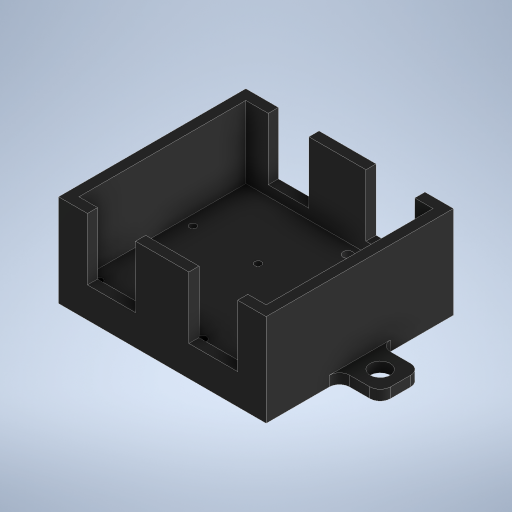
# Autodesk Inventor part: pololuAndRelayCaseBottom
Saved by Autodesk Inventor 2024 (Build 280153000, 153)
## iProperties
Created: 2023-08-11
Part Number: pololuAndRelayCaseBottom
Material: Rubber, Silicone
Document SubType Name: Modeling
Designer: 18179
Density: 1.25 g/cm^3
Appearance: Rubber - Black
Autodesk Inventor part; units mm, degrees
ref_plane "YZ Plane" through (0, 0, 0) normal (1, 0, 0) x (0, 1, 0)
ref_plane "XZ Plane" through (0, 0, 0) normal (0, 1, 0) x (-1, 0, 0)
ref_plane "XY Plane" through (0, 0, 0) normal (0, 0, 1) x (1, 0, 0)
sketch "0" plane through (0, 0, 0) normal (0, 0, 1) x (1, 0, 0)
  line L0 (-1.8843, 38.1841) -> (-1.8843, 30.5641)
  line L1 (-1.8843, 30.5641) -> (-4.4243, 30.5641)
  line L2 (-4.4243, 30.5641) -> (-4.4243, 38.1841)
  line L3 (-4.4243, 38.1841) -> (-1.8843, 38.1841)
  line L4 (0, 50.8) -> (-25.4, 50.8)
  line L5 (-25.4, 50.8) -> (-25.4, 0)
  line L6 (-25.4, 0) -> (0, 0)
  line L7 (0, 0) -> (0, 50.8)
  line L8 (-20.2946, 10.414) -> (-20.2946, 28.194)
  line L9 (-20.2946, 28.194) -> (-5.1054, 28.194)
  line L10 (-5.1054, 28.194) -> (-5.1054, 10.414)
  line L11 (-5.1054, 10.414) -> (-5.08, 10.414)
  line L12 (-5.08, 10.414) -> (-5.08, 2.667)
  line L13 (-5.08, 2.667) -> (-20.32, 2.667)
  line L14 (-20.32, 2.667) -> (-20.32, 10.414)
  line L15 (-20.32, 10.414) -> (-20.2946, 10.414)
  line L16 (-20.32, 41.275) -> (-20.32, 49.022)
  line L17 (-20.32, 49.022) -> (-5.08, 49.022)
  line L18 (-5.08, 49.022) -> (-5.08, 41.275)
  line L19 (-5.08, 41.275) -> (-20.32, 41.275)
  circle A0 centre (-22.733, 2.5852) radius 1.524
  circle A1 centre (-2.667, 2.5852) radius 1.524
  circle A2 centre (-22.733, 48.2148) radius 1.524
  circle A3 centre (-2.667, 48.2148) radius 1.524
  line L20 (-51.95, 5.718) -> (-51.95, 1.218)
  line L21 (-36.95, 1.218) -> (-51.95, 1.218)
  line L22 (-36.95, 5.718) -> (-36.95, 1.218)
  line L23 (-36.95, 5.718) -> (-51.95, 5.718)
  circle A4 centre (-39.45, 3.468) radius 1.775
  circle A5 centre (-44.45, 3.468) radius 1.775
  circle A6 centre (-49.45, 3.468) radius 1.775
  line L24 (-36.95, 7.268) -> (-51.95, 7.268)
  circle A7 centre (-34.29, 2.54) radius 1.0922
  circle A8 centre (-54.61, 2.54) radius 1.0922
  circle A9 centre (-54.61, 31.75) radius 1.0922
  circle A10 centre (-34.29, 31.75) radius 1.0922
  line L25 (-48.655, 31.516) -> (-48.28, 32.141)
  line L26 (-48.28, 32.141) -> (-48.24, 32.141)
  line L27 (-48.24, 32.141) -> (-47.865, 31.516)
  line L28 (-47.865, 31.516) -> (-46.115, 31.516)
  line L29 (-46.115, 31.516) -> (-45.74, 32.141)
  line L30 (-45.74, 32.141) -> (-45.7, 32.141)
  line L31 (-45.7, 32.141) -> (-45.325, 31.516)
  line L32 (-45.325, 31.516) -> (-43.575, 31.516)
  line L33 (-43.575, 31.516) -> (-43.2, 32.141)
  line L34 (-43.2, 32.141) -> (-43.16, 32.141)
  line L35 (-43.16, 32.141) -> (-42.785, 31.516)
  line L36 (-42.785, 31.516) -> (-41.035, 31.516)
  line L37 (-41.035, 31.516) -> (-40.66, 32.141)
  line L38 (-40.66, 32.141) -> (-40.62, 32.141)
  line L39 (-40.62, 32.141) -> (-40.245, 31.516)
  line L40 (-40.245, 31.516) -> (-38.495, 31.516)
  line L41 (-38.495, 31.516) -> (-38.12, 32.141)
  line L42 (-38.12, 32.141) -> (-38.1, 32.141)
  line L43 (-38.1, 32.141) -> (-38.1, 33.391)
  line L44 (-38.1, 33.391) -> (-38.12, 33.391)
  line L45 (-38.12, 33.391) -> (-38.495, 34.016)
  line L46 (-38.495, 34.016) -> (-40.245, 34.016)
  line L47 (-40.245, 34.016) -> (-40.62, 33.391)
  line L48 (-40.62, 33.391) -> (-40.66, 33.391)
  line L49 (-40.66, 33.391) -> (-41.035, 34.016)
  line L50 (-41.035, 34.016) -> (-42.785, 34.016)
  line L51 (-42.785, 34.016) -> (-43.16, 33.391)
  line L52 (-43.16, 33.391) -> (-43.2, 33.391)
  line L53 (-43.2, 33.391) -> (-43.575, 34.016)
  line L54 (-43.575, 34.016) -> (-45.325, 34.016)
  line L55 (-45.325, 34.016) -> (-45.7, 33.391)
  line L56 (-45.7, 33.391) -> (-45.74, 33.391)
  line L57 (-45.74, 33.391) -> (-46.115, 34.016)
  line L58 (-46.115, 34.016) -> (-47.865, 34.016)
  line L59 (-47.865, 34.016) -> (-48.24, 33.391)
  line L60 (-48.24, 33.391) -> (-48.28, 33.391)
  line L61 (-48.28, 33.391) -> (-48.655, 34.016)
  line L62 (-48.655, 34.016) -> (-50.405, 34.016)
  line L63 (-50.405, 34.016) -> (-50.78, 33.391)
  line L64 (-50.78, 33.391) -> (-50.8, 33.391)
  line L65 (-50.8, 33.391) -> (-50.8, 32.141)
  line L66 (-50.8, 32.141) -> (-50.78, 32.141)
  line L67 (-50.78, 32.141) -> (-50.405, 31.516)
  line L68 (-50.405, 31.516) -> (-48.655, 31.516)
  line L69 (-49.205, 32.441) -> (-49.205, 33.091)
  line L70 (-49.205, 32.441) -> (-49.855, 32.441)
  line L71 (-49.855, 32.441) -> (-49.855, 33.091)
  line L72 (-49.205, 33.091) -> (-49.855, 33.091)
  line L73 (-44.125, 32.441) -> (-44.125, 33.091)
  line L74 (-44.125, 32.441) -> (-44.775, 32.441)
  line L75 (-44.775, 32.441) -> (-44.775, 33.091)
  line L76 (-44.125, 33.091) -> (-44.775, 33.091)
  line L77 (-39.045, 32.441) -> (-39.045, 33.091)
  line L78 (-39.045, 32.441) -> (-39.695, 32.441)
  line L79 (-39.695, 32.441) -> (-39.695, 33.091)
  line L80 (-39.045, 33.091) -> (-39.695, 33.091)
  line L81 (-41.585, 32.441) -> (-41.585, 33.091)
  line L82 (-41.585, 32.441) -> (-42.235, 32.441)
  line L83 (-42.235, 32.441) -> (-42.235, 33.091)
  line L84 (-41.585, 33.091) -> (-42.235, 33.091)
  line L85 (-46.665, 32.441) -> (-46.665, 33.091)
  line L86 (-46.665, 32.441) -> (-47.315, 32.441)
  line L87 (-47.315, 32.441) -> (-47.315, 33.091)
  line L88 (-46.665, 33.091) -> (-47.315, 33.091)
  line L89 (-31.75, 34.29) -> (-57.15, 34.29)
  line L90 (-57.15, 34.29) -> (-57.15, 0)
  line L91 (-57.15, 0) -> (-31.75, 0)
  line L92 (-31.75, 0) -> (-31.75, 34.29)
  line L93 (-43.3742, 24.6136) -> (-43.3742, 24.6236)
  line L94 (-43.3742, 24.6236) -> (-42.8742, 24.6236)
  line L95 (-42.8742, 24.6236) -> (-42.8742, 24.6136)
  line L96 (-43.3742, 24.6136) -> (-42.8742, 24.6136)
  line L97 (-42.4242, 24.6136) -> (-42.4242, 24.6236)
  line L98 (-42.4242, 24.6236) -> (-41.9242, 24.6236)
  line L99 (-41.9242, 24.6236) -> (-41.9242, 24.6136)
  line L100 (-42.4242, 24.6136) -> (-41.9242, 24.6136)
  line L101 (-41.4742, 24.6136) -> (-41.4742, 24.6236)
  line L102 (-41.4742, 24.6236) -> (-40.9742, 24.6236)
  line L103 (-40.9742, 24.6236) -> (-40.9742, 24.6136)
  line L104 (-41.4742, 24.6136) -> (-40.9742, 24.6136)
  line L105 (-48.714, 27.3595) -> (-48.714, 27.171)
  line L106 (-48.714, 27.3595) -> (-48.314, 27.3595)
  line L107 (-48.314, 27.3595) -> (-48.314, 27.171)
  line L108 (-48.314, 27.171) -> (-48.714, 27.171)
  line L109 (-48.314, 24.6595) -> (-48.314, 24.848)
  line L110 (-48.714, 24.6595) -> (-48.314, 24.6595)
  line L111 (-48.714, 24.6595) -> (-48.714, 24.848)
  line L112 (-48.714, 24.848) -> (-48.314, 24.848)
  line L113 (-51.0762, 27.3595) -> (-51.0762, 27.171)
  line L114 (-51.0762, 27.3595) -> (-50.6762, 27.3595)
  line L115 (-50.6762, 27.3595) -> (-50.6762, 27.171)
  line L116 (-50.6762, 27.171) -> (-51.0762, 27.171)
  line L117 (-50.6762, 24.6595) -> (-50.6762, 24.848)
  line L118 (-51.0762, 24.6595) -> (-50.6762, 24.6595)
  line L119 (-51.0762, 24.6595) -> (-51.0762, 24.848)
  line L120 (-51.0762, 24.848) -> (-50.6762, 24.848)
  line L121 (-33.109, 6.6231) -> (-33.109, 5.8231)
  line L122 (-33.109, 5.8231) -> (-34.709, 5.8231)
  line L123 (-34.709, 5.8231) -> (-34.709, 6.6231)
  line L124 (-34.709, 6.6231) -> (-33.109, 6.6231)
  line L125 (-47.014, 30.867) -> (-46.714, 30.867)
  line L126 (-46.714, 30.867) -> (-45.614, 30.867)
  line L127 (-45.614, 30.867) -> (-45.314, 30.867)
  line L128 (-45.314, 30.867) -> (-45.314, 29.967)
  line L129 (-45.614, 29.967) -> (-45.314, 29.967)
  line L130 (-45.614, 29.967) -> (-46.714, 29.967)
  line L131 (-47.014, 29.967) -> (-46.714, 29.967)
  line L132 (-47.014, 30.867) -> (-47.014, 29.967)
  line L133 (-47.0018, 29.1022) -> (-46.7018, 29.1022)
  line L134 (-46.7018, 29.1022) -> (-45.6018, 29.1022)
  line L135 (-45.6018, 29.1022) -> (-45.3018, 29.1022)
  line L136 (-45.3018, 29.1022) -> (-45.3018, 28.2022)
  line L137 (-45.6018, 28.2022) -> (-45.3018, 28.2022)
  line L138 (-45.6018, 28.2022) -> (-46.7018, 28.2022)
  line L139 (-47.0018, 28.2022) -> (-46.7018, 28.2022)
  line L140 (-47.0018, 29.1022) -> (-47.0018, 28.2022)
  line L141 (-38.4374, 30.141) -> (-38.4374, 29.041)
  line L142 (-38.4374, 29.041) -> (-38.4374, 28.741)
  line L143 (-38.4374, 28.741) -> (-39.3374, 28.741)
  line L144 (-39.3374, 29.041) -> (-39.3374, 28.741)
  line L145 (-39.3374, 29.041) -> (-39.3374, 30.141)
  line L146 (-39.3374, 30.441) -> (-39.3374, 30.141)
  line L147 (-38.4374, 30.441) -> (-39.3374, 30.441)
  line L148 (-38.4374, 30.441) -> (-38.4374, 30.141)
  line L149 (-34.164, 25.019) -> (-33.654, 25.019)
  line L150 (-34.164, 25.029) -> (-34.164, 25.019)
  line L151 (-34.164, 25.029) -> (-33.654, 25.029)
  line L152 (-33.654, 25.019) -> (-33.654, 25.029)
  line L153 (-34.569, 27.519) -> (-35.079, 27.519)
  line L154 (-34.569, 27.519) -> (-34.569, 27.509)
  line L155 (-34.569, 27.509) -> (-35.079, 27.509)
  line L156 (-35.079, 27.519) -> (-35.079, 27.509)
  line L157 (-32.739, 27.519) -> (-33.249, 27.519)
  line L158 (-32.739, 27.519) -> (-32.739, 27.509)
  line L159 (-32.739, 27.509) -> (-33.249, 27.509)
  line L160 (-33.249, 27.519) -> (-33.249, 27.509)
  line L161 (-48.862, 30.466) -> (-47.912, 30.466)
  line L162 (-47.912, 30.466) -> (-47.912, 28.716)
  line L163 (-47.912, 28.716) -> (-48.862, 28.716)
  line L164 (-48.862, 28.716) -> (-48.862, 30.466)
  line L165 (-40.988, 30.466) -> (-40.038, 30.466)
  line L166 (-40.038, 30.466) -> (-40.038, 28.716)
  line L167 (-40.038, 28.716) -> (-40.988, 28.716)
  line L168 (-40.988, 28.716) -> (-40.988, 30.466)
  line L169 (-42.385, 30.466) -> (-41.435, 30.466)
  line L170 (-41.435, 30.466) -> (-41.435, 28.716)
  line L171 (-41.435, 28.716) -> (-42.385, 28.716)
  line L172 (-42.385, 28.716) -> (-42.385, 30.466)
  line L173 (-37.324, 28.354) -> (-37.324, 29.304)
  line L174 (-37.324, 29.304) -> (-35.574, 29.304)
  line L175 (-35.574, 29.304) -> (-35.574, 28.354)
  line L176 (-35.574, 28.354) -> (-37.324, 28.354)
  line L177 (-50.4114, 30.466) -> (-49.4614, 30.466)
  line L178 (-49.4614, 30.466) -> (-49.4614, 28.716)
  line L179 (-49.4614, 28.716) -> (-50.4114, 28.716)
  line L180 (-50.4114, 28.716) -> (-50.4114, 30.466)
  line L181 (-55.612, 24.671) -> (-55.612, 25.621)
  line L182 (-55.612, 25.621) -> (-53.862, 25.621)
  line L183 (-53.862, 25.621) -> (-53.862, 24.671)
  line L184 (-53.862, 24.671) -> (-55.612, 24.671)
  line L185 (-43.7312, 30.466) -> (-42.7812, 30.466)
  line L186 (-42.7812, 30.466) -> (-42.7812, 28.716)
  line L187 (-42.7812, 28.716) -> (-43.7312, 28.716)
  line L188 (-43.7312, 28.716) -> (-43.7312, 30.466)
  line L189 (-41.4742, 27.558) -> (-40.9742, 27.558)
  line L190 (-40.9742, 27.548) -> (-40.9742, 27.558)
  line L191 (-41.4742, 27.548) -> (-40.9742, 27.548)
  line L192 (-41.4742, 27.558) -> (-41.4742, 27.548)
  line L193 (-42.4242, 27.558) -> (-41.9242, 27.558)
  line L194 (-41.9242, 27.548) -> (-41.9242, 27.558)
  line L195 (-42.4242, 27.548) -> (-41.9242, 27.548)
  line L196 (-42.4242, 27.558) -> (-42.4242, 27.548)
  line L197 (-43.3742, 27.558) -> (-42.8742, 27.558)
  line L198 (-42.8742, 27.548) -> (-42.8742, 27.558)
  line L199 (-43.3742, 27.548) -> (-42.8742, 27.548)
  line L200 (-43.3742, 27.558) -> (-43.3742, 27.548)
  line L201 (-38.9509, 26.6649) -> (-38.9509, 26.1671)
  line L202 (-38.9409, 26.6649) -> (-38.9509, 26.6649)
  line L203 (-38.9409, 26.6649) -> (-38.9409, 26.1671)
  line L204 (-38.9509, 26.1671) -> (-38.9409, 26.1671)
  line L205 (-38.9509, 27.6174) -> (-38.9509, 27.1196)
  line L206 (-38.9409, 27.6174) -> (-38.9509, 27.6174)
  line L207 (-38.9409, 27.6174) -> (-38.9409, 27.1196)
  line L208 (-38.9509, 27.1196) -> (-38.9409, 27.1196)
  line L209 (-38.9509, 25.7124) -> (-38.9509, 25.2146)
  line L210 (-38.9409, 25.7124) -> (-38.9509, 25.7124)
  line L211 (-38.9409, 25.7124) -> (-38.9409, 25.2146)
  line L212 (-38.9509, 25.2146) -> (-38.9409, 25.2146)
  line L213 (-35.9637, 27.6174) -> (-35.9637, 27.1196)
  line L214 (-35.9537, 27.6174) -> (-35.9637, 27.6174)
  line L215 (-35.9537, 27.6174) -> (-35.9537, 27.1196)
  line L216 (-35.9637, 27.1196) -> (-35.9537, 27.1196)
  line L217 (-35.9637, 25.7124) -> (-35.9637, 25.2146)
  line L218 (-35.9537, 25.7124) -> (-35.9637, 25.7124)
  line L219 (-35.9537, 25.7124) -> (-35.9537, 25.2146)
  line L220 (-35.9637, 25.2146) -> (-35.9537, 25.2146)
  line L221 (-45.9984, 27.3304) -> (-46.5084, 27.3304)
  line L222 (-45.9984, 27.3204) -> (-45.9984, 27.3304)
  line L223 (-45.9984, 27.3204) -> (-46.5084, 27.3204)
  line L224 (-46.5084, 27.3304) -> (-46.5084, 27.3204)
  line L225 (-45.5934, 24.8304) -> (-45.0834, 24.8304)
  line L226 (-45.5934, 24.8304) -> (-45.5934, 24.8404)
  line L227 (-45.5934, 24.8404) -> (-45.0834, 24.8404)
  line L228 (-45.0834, 24.8304) -> (-45.0834, 24.8404)
  line L229 (-47.4234, 24.8304) -> (-46.9134, 24.8304)
  line L230 (-47.4234, 24.8304) -> (-47.4234, 24.8404)
  line L231 (-47.4234, 24.8404) -> (-46.9134, 24.8404)
  line L232 (-46.9134, 24.8304) -> (-46.9134, 24.8404)
  circle A11 centre (-53.0606, 27.8892) radius 0.508
  circle A12 centre (-44.45, 3.068) radius 0.889
  circle A13 centre (-39.45, 3.068) radius 0.889
  circle A14 centre (-49.45, 3.068) radius 0.889
  circle A15 centre (-39.37, 32.766) radius 0.508
  circle A16 centre (-55.6006, 27.8892) radius 0.508
  circle A17 centre (-50.324, 21.748) radius 0.762
  circle A18 centre (-38.124, 21.748) radius 0.762
  circle A19 centre (-38.124, 9.748) radius 0.762
  circle A20 centre (-50.324, 9.748) radius 0.762
  circle A21 centre (-52.324, 15.748) radius 0.762
  circle A22 centre (-54.61, 31.75) radius 1.0922
  circle A23 centre (-34.29, 31.75) radius 1.0922
  circle A24 centre (-54.61, 2.54) radius 1.0922
  circle A25 centre (-49.53, 4.826) radius 0.508
  circle A26 centre (-44.45, 4.826) radius 0.508
  circle A27 centre (-41.91, 32.766) radius 0.508
  circle A28 centre (-44.45, 32.766) radius 0.508
  circle A29 centre (-46.99, 32.766) radius 0.508
  circle A30 centre (-49.53, 32.766) radius 0.508
  circle A31 centre (-34.29, 2.54) radius 1.0922
  circle A32 centre (-39.37, 4.826) radius 0.508
  line L233 (-25.4, 0) -> (-31.75, 0)
  line L234 (-31.75, 0) -> (-31.75, 12.7114)
  line L235 (-31.75, 12.7114) -> (-25.4, 12.7114)
  line L236 (-25.4, 12.7114) -> (-25.4, 0)
  point P0 (-57.15, 34.29)
  dimension "d0" = 6.35
  constraints: 474 end point, 33 centre point, 2 parallel, 1 horizontal, 1 perpendicular
  measures "d0" distance of L234.end L235.end
extrude "Extrusion1" add sketch "0" along normal blind 3.175 contours L0 L1 L2 L3 | L7 L6 L5 L4 | L92 L91 L90 L89 | L93 L94 L95 L96 | L97 L98 L99 L100 | L101 L102 L103 L104 | L106 L107 L108 L105 | L110 L111 L112 L109 | L114 L115 L116 L113 | L118 L119 L120 L117 | L121 L122 L123 L124 | L125 L126 L127 L128 L129 L130 L131 L132 | L133 L134 L135 L136 L137 L138 L139 L140 | L141 L142 L143 L144 L145 L146 L147 L148 | L150 L151 L152 L149 | L154 L155 L156 L153 | L161 L162 L163 L164 | L165 L166 L167 L168 | L169 L170 L171 L172 | L173 L174 L175 L176 | L177 L178 L179 L180 | L181 L182 L183 L184 | L185 L186 L187 L188 | L189 L190 L191 L192 | L193 L194 L195 L196 | L197 L198 L199 L200 | L202 L203 L204 L201 | L206 L207 L208 L205 | L210 L211 L212 L209 | L214 L215 L216 L213 | L218 L219 L220 L217 | L222 L223 L224 L221 | L226 L227 L228 L225 | L230 L231 L232 L229 | A11 | A16 | A17 | A18 | A19 | A20 | A21
sketch "Sketch3" plane through (0, 0, 3.175) normal (0, 0, 1) x (1, 0, 0)
  line L0 (-57.15, 34.29) -> (-57.15, 0) projected
  line L1 (0, 0) -> (0, 50.8) projected
  line L2 (-57.15, 0) -> (0, 0)
  line L3 (0, 0) -> (0, 50.8)
  line L4 (0, 50.8) -> (-57.15, 50.8)
  line L5 (-57.15, 50.8) -> (-57.15, 0)
  line L6 (-57.785, 51.435) -> (0.635, 51.435)
  line L7 (0.635, 51.435) -> (0.635, -0.635)
  line L8 (0.635, -0.635) -> (-57.785, -0.635)
  line L9 (-57.785, -0.635) -> (-57.785, 51.435)
  line L10 (3.81, 54.61) -> (-60.96, 54.61)
  line L11 (-60.96, 54.61) -> (-60.96, -3.81)
  line L12 (-60.96, -3.81) -> (3.81, -3.81)
  line L13 (3.81, -3.81) -> (3.81, 54.61)
  dimension "d3" = 0.635
  dimension "d4" = 3.175
  constraints: 24 end point, 6 parallel, 3 perpendicular, 1 horizontal, 6 other
  measures "d3" distance between parallel lines of L4 L6
  measures "d4" distance between parallel lines of L6 L10
extrude "Extrusion2" add sketch "Sketch3" along normal blind 3.175 contours L13 L12 L11 L10
sketch "Sketch4" plane through (0, 0, 6.35) normal (0, 0, 1) x (1, 0, 0)
  line L0 (-31.75, 0) -> (-31.75, 34.29) projected
  line L1 (-31.75, 34.29) -> (-57.15, 34.29) projected
  line L2 (-57.15, 34.29) -> (-57.15, 0) projected
  line L3 (-57.15, 0) -> (-31.75, 0) projected
  line L4 (-36.95, 5.718) -> (-36.95, 1.218) projected
  line L5 (-36.95, 1.218) -> (-51.95, 1.218) projected
  line L6 (-51.95, 1.218) -> (-51.95, 5.718) projected
  line L7 (-51.95, 5.718) -> (-36.95, 5.718) projected
  line L8 (-48.655, 31.516) -> (-50.405, 31.516) projected
  line L9 (-50.405, 31.516) -> (-50.78, 32.141) projected
  line L10 (-50.78, 32.141) -> (-50.8, 32.141) projected
  line L11 (-50.8, 32.141) -> (-50.8, 33.391) projected
  line L12 (-50.8, 33.391) -> (-50.78, 33.391) projected
  line L13 (-50.78, 33.391) -> (-50.405, 34.016) projected
  line L14 (-50.405, 34.016) -> (-48.655, 34.016) projected
  line L15 (-48.655, 34.016) -> (-48.28, 33.391) projected
  line L16 (-48.28, 33.391) -> (-48.24, 33.391) projected
  line L17 (-48.24, 33.391) -> (-47.865, 34.016) projected
  line L18 (-47.865, 34.016) -> (-46.115, 34.016) projected
  line L19 (-46.115, 34.016) -> (-45.74, 33.391) projected
  line L20 (-45.74, 33.391) -> (-45.7, 33.391) projected
  line L21 (-45.7, 33.391) -> (-45.325, 34.016) projected
  line L22 (-45.325, 34.016) -> (-43.575, 34.016) projected
  line L23 (-43.575, 34.016) -> (-43.2, 33.391) projected
  line L24 (-43.2, 33.391) -> (-43.16, 33.391) projected
  line L25 (-43.16, 33.391) -> (-42.785, 34.016) projected
  line L26 (-42.785, 34.016) -> (-41.035, 34.016) projected
  line L27 (-41.035, 34.016) -> (-40.66, 33.391) projected
  line L28 (-40.66, 33.391) -> (-40.62, 33.391) projected
  line L29 (-40.62, 33.391) -> (-40.245, 34.016) projected
  line L30 (-40.245, 34.016) -> (-38.495, 34.016) projected
  line L31 (-38.495, 34.016) -> (-38.12, 33.391) projected
  line L32 (-38.12, 33.391) -> (-38.1, 33.391) projected
  line L33 (-38.1, 33.391) -> (-38.1, 32.141) projected
  line L34 (-38.1, 32.141) -> (-38.12, 32.141) projected
  line L35 (-38.12, 32.141) -> (-38.495, 31.516) projected
  line L36 (-38.495, 31.516) -> (-40.245, 31.516) projected
  line L37 (-40.245, 31.516) -> (-40.62, 32.141) projected
  line L38 (-40.62, 32.141) -> (-40.66, 32.141) projected
  line L39 (-40.66, 32.141) -> (-41.035, 31.516) projected
  line L40 (-41.035, 31.516) -> (-42.785, 31.516) projected
  line L41 (-42.785, 31.516) -> (-43.16, 32.141) projected
  line L42 (-43.16, 32.141) -> (-43.2, 32.141) projected
  line L43 (-43.2, 32.141) -> (-43.575, 31.516) projected
  line L44 (-43.575, 31.516) -> (-45.325, 31.516) projected
  line L45 (-45.325, 31.516) -> (-45.7, 32.141) projected
  line L46 (-45.7, 32.141) -> (-45.74, 32.141) projected
  line L47 (-45.74, 32.141) -> (-46.115, 31.516) projected
  line L48 (-46.115, 31.516) -> (-47.865, 31.516) projected
  line L49 (-47.865, 31.516) -> (-48.24, 32.141) projected
  line L50 (-48.24, 32.141) -> (-48.28, 32.141) projected
  line L51 (-48.28, 32.141) -> (-48.655, 31.516) projected
  line L52 (-32.739, 27.509) -> (-33.249, 27.509) projected
  line L53 (-33.249, 27.509) -> (-33.249, 27.519) projected
  line L54 (-33.249, 27.519) -> (-32.739, 27.519) projected
  line L55 (-32.739, 27.519) -> (-32.739, 27.509) projected
  circle A0 centre (-54.61, 31.75) radius 1.0922 projected
  circle A1 centre (-34.29, 2.54) radius 1.0922 projected
  circle A2 centre (-54.61, 2.54) radius 1.0922 projected
  circle A3 centre (-34.29, 31.75) radius 1.0922 projected
  line L56 (-25.4, 50.8) -> (-25.4, 0) projected
  line L57 (-25.4, 0) -> (0, 0) projected
  line L58 (0, 0) -> (0, 50.8) projected
  line L59 (0, 50.8) -> (-25.4, 50.8) projected
  circle A4 centre (-2.667, 48.2148) radius 1.524 projected
  circle A5 centre (-22.733, 48.2148) radius 1.524 projected
  circle A6 centre (-2.667, 2.5852) radius 1.524 projected
  circle A7 centre (-22.733, 2.5852) radius 1.524 projected
  line L60 (-20.32, 41.275) -> (-20.32, 49.022) projected
  line L61 (-20.32, 49.022) -> (-5.08, 49.022) projected
  line L62 (-5.08, 49.022) -> (-5.08, 41.275) projected
  line L63 (-5.08, 41.275) -> (-20.32, 41.275) projected
  line L64 (-20.2946, 10.414) -> (-20.2946, 28.194) projected
  line L65 (-20.2946, 28.194) -> (-5.1054, 28.194) projected
  line L66 (-5.1054, 28.194) -> (-5.1054, 10.414) projected
  line L67 (-5.1054, 10.414) -> (-5.08, 10.414) projected
  line L68 (-5.08, 10.414) -> (-5.08, 2.667) projected
  line L69 (-5.08, 2.667) -> (-20.32, 2.667) projected
  line L70 (-20.32, 2.667) -> (-20.32, 10.414) projected
  line L71 (-20.32, 10.414) -> (-20.2946, 10.414) projected
  line L72 (-60.96, 54.61) -> (-60.96, -3.81) projected
  line L73 (-60.96, -3.81) -> (3.81, -3.81) projected
  line L74 (3.81, -3.81) -> (3.81, 54.61) projected
  line L75 (3.81, 54.61) -> (-60.96, 54.61) projected
  line L76 (-57.785, 51.435) -> (0.635, 51.435) projected
  line L77 (0.635, 51.435) -> (0.635, -0.635) projected
  line L78 (0.635, -0.635) -> (-57.785, -0.635) projected
  line L79 (-57.785, -0.635) -> (-57.785, 51.435) projected
  line L80 (-51.95, 1.218) -> (-36.95, 1.218)
  line L81 (-36.95, 1.218) -> (-36.95, -3.81)
  line L82 (-36.95, -3.81) -> (-51.95, -3.81)
  line L83 (-51.95, -3.81) -> (-51.95, 1.218)
  line L84 (-20.32, 2.667) -> (-5.08, 2.667)
  line L85 (-5.08, 2.667) -> (-5.08, -3.81)
  line L86 (-5.08, -3.81) -> (-20.32, -3.81)
  line L87 (-20.32, -3.81) -> (-20.32, 2.667)
  line L88 (-5.08, 49.022) -> (-20.32, 49.022)
  line L89 (-20.32, 49.022) -> (-20.32, 54.61)
  line L90 (-20.32, 54.61) -> (-5.08, 54.61)
  line L91 (-5.08, 54.61) -> (-5.08, 49.022)
  line L92 (-50.8, 32.141) -> (-38.12, 32.141)
  line L93 (-38.12, 32.141) -> (-38.12, 54.61)
  line L94 (-38.12, 54.61) -> (-50.8, 54.61)
  line L95 (-50.8, 54.61) -> (-50.8, 32.141)
  point P0 (-20.32, -0.635)
  point P1 (-36.95, -0.635)
  point P2 (-5.08, 51.435)
  point P3 (-5.08, -0.635)
  point P4 (-38.12, 51.435)
  point P5 (-20.32, 51.435)
  point P6 (-51.95, -0.635)
  point P7 (-50.8, 51.435)
  constraints: 32 end point, 8 parallel, 5 point on line, 4 horizontal, 4 perpendicular
extrude "Extrusion3" add sketch "Sketch4" along normal blind 19.304 contours L78 L87 L73 L81 | L93 L75 L89 L76 | L83 L73 L72 L75 L95 L76 L79 L78 | L78 L77 L76 L91 L75 L74 L73 L85
sketch "Sketch5" plane through (0, 0, 3.175) normal (0, 0, 1) x (1, 0, 0)
  line L0 (-31.75, 0) -> (-31.75, 34.29) projected
  line L1 (-31.75, 34.29) -> (-57.15, 34.29) projected
  line L2 (-57.15, 34.29) -> (-57.15, 0) projected
  line L3 (-57.15, 0) -> (-31.75, 0) projected
  line L4 (-36.95, 5.718) -> (-36.95, 1.218) projected
  line L5 (-36.95, 1.218) -> (-51.95, 1.218) projected
  line L6 (-51.95, 1.218) -> (-51.95, 5.718) projected
  line L7 (-51.95, 5.718) -> (-36.95, 5.718) projected
  line L8 (-48.655, 31.516) -> (-50.405, 31.516) projected
  line L9 (-50.405, 31.516) -> (-50.78, 32.141) projected
  line L10 (-50.78, 32.141) -> (-50.8, 32.141) projected
  line L11 (-50.8, 32.141) -> (-50.8, 33.391) projected
  line L12 (-50.8, 33.391) -> (-50.78, 33.391) projected
  line L13 (-50.78, 33.391) -> (-50.405, 34.016) projected
  line L14 (-50.405, 34.016) -> (-48.655, 34.016) projected
  line L15 (-48.655, 34.016) -> (-48.28, 33.391) projected
  line L16 (-48.28, 33.391) -> (-48.24, 33.391) projected
  line L17 (-48.24, 33.391) -> (-47.865, 34.016) projected
  line L18 (-47.865, 34.016) -> (-46.115, 34.016) projected
  line L19 (-46.115, 34.016) -> (-45.74, 33.391) projected
  line L20 (-45.74, 33.391) -> (-45.7, 33.391) projected
  line L21 (-45.7, 33.391) -> (-45.325, 34.016) projected
  line L22 (-45.325, 34.016) -> (-43.575, 34.016) projected
  line L23 (-43.575, 34.016) -> (-43.2, 33.391) projected
  line L24 (-43.2, 33.391) -> (-43.16, 33.391) projected
  line L25 (-43.16, 33.391) -> (-42.785, 34.016) projected
  line L26 (-42.785, 34.016) -> (-41.035, 34.016) projected
  line L27 (-41.035, 34.016) -> (-40.66, 33.391) projected
  line L28 (-40.66, 33.391) -> (-40.62, 33.391) projected
  line L29 (-40.62, 33.391) -> (-40.245, 34.016) projected
  line L30 (-40.245, 34.016) -> (-38.495, 34.016) projected
  line L31 (-38.495, 34.016) -> (-38.12, 33.391) projected
  line L32 (-38.12, 33.391) -> (-38.1, 33.391) projected
  line L33 (-38.1, 33.391) -> (-38.1, 32.141) projected
  line L34 (-38.1, 32.141) -> (-38.12, 32.141) projected
  line L35 (-38.12, 32.141) -> (-38.495, 31.516) projected
  line L36 (-38.495, 31.516) -> (-40.245, 31.516) projected
  line L37 (-40.245, 31.516) -> (-40.62, 32.141) projected
  line L38 (-40.62, 32.141) -> (-40.66, 32.141) projected
  line L39 (-40.66, 32.141) -> (-41.035, 31.516) projected
  line L40 (-41.035, 31.516) -> (-42.785, 31.516) projected
  line L41 (-42.785, 31.516) -> (-43.16, 32.141) projected
  line L42 (-43.16, 32.141) -> (-43.2, 32.141) projected
  line L43 (-43.2, 32.141) -> (-43.575, 31.516) projected
  line L44 (-43.575, 31.516) -> (-45.325, 31.516) projected
  line L45 (-45.325, 31.516) -> (-45.7, 32.141) projected
  line L46 (-45.7, 32.141) -> (-45.74, 32.141) projected
  line L47 (-45.74, 32.141) -> (-46.115, 31.516) projected
  line L48 (-46.115, 31.516) -> (-47.865, 31.516) projected
  line L49 (-47.865, 31.516) -> (-48.24, 32.141) projected
  line L50 (-48.24, 32.141) -> (-48.28, 32.141) projected
  line L51 (-48.28, 32.141) -> (-48.655, 31.516) projected
  line L52 (-32.739, 27.509) -> (-33.249, 27.509) projected
  line L53 (-33.249, 27.509) -> (-33.249, 27.519) projected
  line L54 (-33.249, 27.519) -> (-32.739, 27.519) projected
  line L55 (-32.739, 27.519) -> (-32.739, 27.509) projected
  circle A0 centre (-54.61, 31.75) radius 1.0922 projected
  circle A1 centre (-34.29, 2.54) radius 1.0922 projected
  circle A2 centre (-54.61, 2.54) radius 1.0922 projected
  circle A3 centre (-34.29, 31.75) radius 1.0922 projected
  line L56 (-25.4, 50.8) -> (-25.4, 0) projected
  line L57 (-25.4, 0) -> (0, 0) projected
  line L58 (0, 0) -> (0, 50.8) projected
  line L59 (0, 50.8) -> (-25.4, 50.8) projected
  circle A4 centre (-2.667, 48.2148) radius 1.524 projected
  circle A5 centre (-22.733, 48.2148) radius 1.524 projected
  circle A6 centre (-2.667, 2.5852) radius 1.524 projected
  circle A7 centre (-22.733, 2.5852) radius 1.524 projected
  line L60 (-20.32, 41.275) -> (-20.32, 49.022) projected
  line L61 (-20.32, 49.022) -> (-5.08, 49.022) projected
  line L62 (-5.08, 49.022) -> (-5.08, 41.275) projected
  line L63 (-5.08, 41.275) -> (-20.32, 41.275) projected
  line L64 (-20.2946, 10.414) -> (-20.2946, 28.194) projected
  line L65 (-20.2946, 28.194) -> (-5.1054, 28.194) projected
  line L66 (-5.1054, 28.194) -> (-5.1054, 10.414) projected
  line L67 (-5.1054, 10.414) -> (-5.08, 10.414) projected
  line L68 (-5.08, 10.414) -> (-5.08, 2.667) projected
  line L69 (-5.08, 2.667) -> (-20.32, 2.667) projected
  line L70 (-20.32, 2.667) -> (-20.32, 10.414) projected
  line L71 (-20.32, 10.414) -> (-20.2946, 10.414) projected
  line L72 (3.81, 54.61) -> (-5.08, 54.61) projected
  line L73 (-5.08, 54.61) -> (-5.08, 51.435) projected
  line L74 (-5.08, 51.435) -> (0.635, 51.435) projected
  line L75 (0.635, 51.435) -> (0.635, -0.635) projected
  line L76 (0.635, -0.635) -> (-5.08, -0.635) projected
  line L77 (-5.08, -0.635) -> (-5.08, -3.81) projected
  line L78 (-5.08, -3.81) -> (3.81, -3.81) projected
  line L79 (3.81, -3.81) -> (3.81, 54.61) projected
  line L80 (-60.96, -3.81) -> (-51.95, -3.81) projected
  line L81 (-51.95, -3.81) -> (-51.95, -0.635) projected
  line L82 (-51.95, -0.635) -> (-57.785, -0.635) projected
  line L83 (-57.785, -0.635) -> (-57.785, 51.435) projected
  line L84 (-57.785, 51.435) -> (-50.8, 51.435) projected
  line L85 (-50.8, 51.435) -> (-50.8, 54.61) projected
  line L86 (-50.8, 54.61) -> (-60.96, 54.61) projected
  line L87 (-60.96, 54.61) -> (-60.96, -3.81) projected
  line L88 (-60.96, 54.61) -> (-60.96, -3.81) projected
  line L89 (-60.96, 54.61) -> (3.81, 54.61)
  line L90 (3.81, 54.61) -> (3.81, -3.81)
  line L91 (3.81, -3.81) -> (-60.96, -3.81)
  line L92 (-60.96, -3.81) -> (-60.96, 54.61)
  constraints: 8 end point, 2 parallel, 1 horizontal, 1 perpendicular
extrude "Extrusion4" add sketch "Sketch5" against normal blind 3.175 contours L3 L2 L1 L0 | L4 L5 L6 L7 | L8 L9 L10 L11 L12 L13 L14 L15 L16 L17 L18 L19 L20 L21 L22 L23 L24 L25 L26 L27 L28 L29 L30 L31 L32 L33 L34 L35 L36 L37 L38 L39 L40 L41 L42 L43 L44 L45 L46 L47 L48 L49 L50 L51 | L52 L53 L54 L55 | L59 L58 L57 L56 | L60 L61 L62 L63 | L64 L65 L66 L67 L68 L69 L70 L71 | L79 L78 L77 L76 L75 L74 L73 L72 | L73 L74 L75 L76 L77 L91 L81 L82 L83 L84 L85 L89 | L85 L84 L83 L82 L81 L80 L87 L86
sketch "Sketch6" plane through (0, 0, 25.654) normal (0, 0, 1) x (1, 0, 0)
  line L0 (-20.32, 51.435) -> (-5.08, 51.435)
  line L1 (-5.08, 51.435) -> (-5.08, 45.847)
  line L2 (-5.08, 45.847) -> (-20.32, 45.847)
  line L3 (-20.32, 45.847) -> (-20.32, 51.435)
  line L4 (-20.32, -0.635) -> (-36.95, -0.635) projected
  line L5 (-20.32, -0.635) -> (-5.08, -0.635)
  line L6 (-5.08, -0.635) -> (-5.08, 4.953)
  line L7 (-5.08, 4.953) -> (-20.32, 4.953)
  line L8 (-20.32, 4.953) -> (-20.32, -0.635)
  line L9 (-36.95, -0.635) -> (-51.95, -0.635)
  line L10 (-51.95, -0.635) -> (-51.95, 4.953)
  line L11 (-51.95, 4.953) -> (-36.95, 4.953)
  line L12 (-36.95, 4.953) -> (-36.95, -0.635)
  line L13 (-50.8, 54.61) -> (-60.96, 54.61) projected
  line L14 (-60.96, 54.61) -> (-60.96, -3.81) projected
  line L15 (-5.08, -3.81) -> (3.81, -3.81) projected
  line L16 (3.81, -3.81) -> (3.81, 54.61) projected
  line L17 (3.81, -3.81) -> (-60.96, -3.81) projected
  line L18 (3.81, -3.81) -> (-60.96, -3.81)
  line L19 (-60.96, -3.81) -> (-60.96, 54.61)
  line L20 (-60.96, 54.61) -> (3.81, 54.61)
  line L21 (3.81, 54.61) -> (3.81, -3.81)
  circle A0 centre (-54.61, 31.75) radius 1.0922 projected
  circle A1 centre (-34.29, 31.75) radius 1.0922 projected
  line L22 (-54.61, 31.75) -> (-34.29, 31.75)
  line L23 (-44.45, 31.75) -> (-50.8, 31.75)
  line L24 (-50.8, 31.75) -> (-50.8, 28.956)
  line L25 (-50.8, 28.956) -> (-44.45, 28.956)
  line L26 (-44.45, 28.956) -> (-44.45, 31.75)
  line L27 (-50.8, 28.956) -> (-38.12, 28.956)
  line L28 (-38.12, 28.956) -> (-38.12, 34.544)
  line L29 (-38.12, 34.544) -> (-50.8, 34.544)
  line L30 (-50.8, 34.544) -> (-50.8, 28.956)
  point P0 (0, 0)
  dimension "d11" = 5.588
  dimension "d12" = 5.588
  dimension "d13" = 5.588
  dimension "d14" = 2.794
  dimension "d15" = 5.588
  constraints: 50 end point, 12 parallel, 7 horizontal, 6 perpendicular, 1 midpoint, 1 point on line
  measures "d11" distance of L0.end L1.end
  measures "d12" distance of L5.end L6.end
  measures "d13" distance of L9.end L10.end
  measures "d14" distance of L24.end L23.end
  measures "d15" distance of L28.end L27.end
sketch "Sketch7" plane through (0, 0, 0) normal (0, 0, -1) x (-1, 0, 0)
  circle A0 centre (34.29, 31.75) radius 1.0922 projected
  circle A1 centre (54.61, 2.54) radius 1.0922 projected
  circle A2 centre (34.29, 2.54) radius 1.0922 projected
  circle A3 centre (54.61, 31.75) radius 1.0922 projected
  line L0 (-3.81, -3.81) -> (60.96, -3.81) projected
  line L1 (60.96, -3.81) -> (60.96, 54.61) projected
  line L2 (60.96, 54.61) -> (-3.81, 54.61) projected
  line L3 (-3.81, 54.61) -> (-3.81, -3.81) projected
  circle A4 centre (2.667, 48.2148) radius 1.524 projected
  circle A5 centre (22.733, 48.2148) radius 1.524 projected
  circle A6 centre (2.667, 2.5852) radius 1.524 projected
  circle A7 centre (22.733, 2.5852) radius 1.524 projected
  line L4 (57.785, -0.635) -> (-0.635, -0.635)
  line L5 (-0.635, -0.635) -> (-0.635, 51.435)
  line L6 (-0.635, 51.435) -> (57.785, 51.435)
  line L7 (57.785, 51.435) -> (57.785, -0.635)
  line L8 (60.96, -3.81) -> (60.96, 54.61) projected
  line L9 (60.96, 25.4) -> (73.66, 25.4)
  line L10 (73.66, 25.4) -> (73.66, 22.225)
  line L11 (70.485, 19.05) -> (60.96, 19.05)
  line L12 (60.96, 19.05) -> (60.96, 25.4)
  line L13 (73.66, 25.4) -> (60.96, 25.4)
  line L14 (60.96, 25.4) -> (60.96, 30.6578)
  line L15 (60.96, 30.6578) -> (70.485, 30.6578)
  line L16 (73.66, 27.4828) -> (73.66, 25.4)
  line L17 (-3.81, 19.05) -> (-13.335, 19.05)
  line L18 (-16.51, 22.225) -> (-16.51, 28.575)
  line L19 (-13.335, 31.75) -> (-3.81, 31.75)
  line L20 (-3.81, 31.75) -> (-3.81, 19.05)
  circle A8 centre (67.31, 25.4) radius 3.175
  circle A9 centre (-10.16, 25.4) radius 3.175
  arc A10 (70.485, 19.05) -> (73.66, 22.225) centre (70.485, 22.225) ccw
  arc A11 (73.66, 27.4828) -> (70.485, 30.6578) centre (70.485, 27.4828) ccw
  arc A12 (-13.335, 31.75) -> (-16.51, 28.575) centre (-13.335, 28.575) ccw
  arc A13 (-16.51, 22.225) -> (-13.335, 19.05) centre (-13.335, 22.225) ccw
  point P0 (0, 0)
  point P1 (73.66, 19.05)
  point P2 (73.66, 30.6578)
  point P3 (-16.51, 31.75)
  point P4 (-16.51, 19.05)
  dimension "d16" = 3.175
  dimension "d17" = 12.7
  dimension "d18" = 6.35
  dimension "d19" = 12.7
  dimension "d20" = 12.7
  dimension "d21" = 12.7
  dimension "d22" = 6.35
  dimension "d23" = 6.35
  dimension "d24" = 3.175
  constraints: 32 end point, 9 point on line, 8 point on circle, 8 tangent, 6 centre point, 6 parallel, 3 equal radius, 3 horizontal, 3 perpendicular, 2 midpoint, 3 other
  measures "d16" distance between parallel lines of L0 L4
  measures "d17" distance of point (73.66, 19.05) L11.end
  measures "d18" distance of L9.end point (73.66, 19.05)
  measures "d19" distance of L14.end point (73.66, 30.658)
  measures "d20" distance of point (-16.51, 31.75) L19.end
  measures "d21" distance of point (-16.51, 19.05) point (-16.51, 31.75)
  measures "d22" diameter of A8
  measures "d23" diameter of A9
  measures "d24" radius of A10
extrude "Extrusion5" add sketch "Sketch7" along normal blind 3.175 contours L3 L2 L1 L0 | L17 A13 L18 A12 L19 L3 | L1 L9 A8 L10 A10 L11 | L1 L15 A11 L16 L9 A8
fillet "Fillet1" radius 3.175 4 edges at (3.81, 19.05, -1.5875) (3.81, 31.75, -1.5875) (-60.96, 30.6578, -1.5875) (-60.96, 19.05, -1.5875)
body "Solid1"
